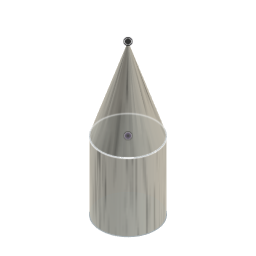
varilla_80mm (Autodesk Fusion 360 design; units mm, degrees)
Autodesk Fusion 360 part; units mm, degrees
sketch "Boceto1" plane through (0, 0, 0) normal (0, 0, 1) x (1, 0, 0)
  circle A0 centre (0, 0) radius 4
  dimension "d1" = 8
  constraint coincident A0.centre origin
  measures "d1" diameter of A0
ref_plane "PlanoDeObra2" through (0, 0, 10) normal (0, 0, 1) x (1, 0, 0)
ref_plane "PlanoDeObra3" through (0, 0, 22) normal (0, 0, 1) x (1, 0, 0)
sketch "Boceto5" plane through (0, 0, 22) normal (0, 0, 1) x (1, 0, 0)
sketch "Boceto6" plane through (0, 0, 10) normal (0, 0, 1) x (1, 0, 0)
  circle A0 centre (0, 0) radius 4
  dimension "d15" = 8
  constraint coincident A0.centre origin
  measures "d15" diameter of A0
loft "Solevación1" add profiles "Boceto6" section 1 point at (0, 0, 22) section 2
extrude "Extruir1" add 1 faces at (-0.9774, 0.9069, 10) along direction (0, 0, -1) blind 10
sketch "Boceto7" plane through (0, 0, 0) normal (0, 0, -1) x (1, 0, 0)
  circle A0 centre (0, 0) radius 4
